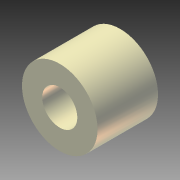
# Autodesk Inventor part: inner_block
Saved by Autodesk Inventor 2011 SP2 (Build 150309200, 309)
## iProperties
Created: 2013-09-16
Part Number: inner_block
Document SubType Name: Modeling
Designer: sungwook
Density: 1 g/cm^3
Author: sungwook
Autodesk Inventor part; units mm, degrees
ref_plane "YZ Plane" through (0, 0, 0) normal (1, 0, 0) x (0, 1, 0)
ref_plane "XZ Plane" through (0, 0, 0) normal (0, 1, 0) x (-1, 0, 0)
ref_plane "XY Plane" through (0, 0, 0) normal (0, 0, 1) x (1, 0, 0)
sketch "Sketch1" plane through (0, 0, 0) normal (0, 0, 1) x (1, 0, 0)
  circle A0 centre (0, 0) radius 1.5875
  dimension "d0" = 3.175
  constraints: 1 centre point, 1 coincident
  measures "d0" diameter of A0
extrude "Extrusion1" add sketch "Sketch1" along normal blind 2.54
hole "Hole1" at (0, 0, 0) direction (0, 0, 1) diameter 1.4732 end through all
body "Solid1"
